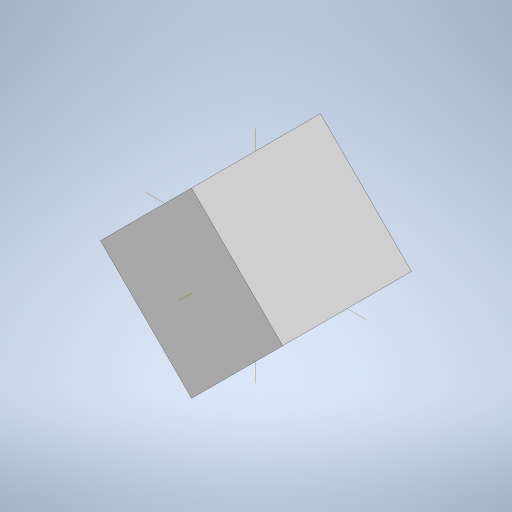
# Autodesk Inventor part: Cube
Saved by Autodesk Inventor 2023.1 (Build 271208000, 208)
## iProperties
Created: 2023-01-19
Part Number: Cube
Material: Generisch
Document SubType Name: Modeling
Designer: mehan
Density: 1 g/cm^3
Appearance: Vorgabe
Author: mehan
Autodesk Inventor part; units mm, degrees
ref_plane "YZ Plane" through (0, 0, 0) normal (1, 0, 0) x (0, 1, 0)
ref_plane "XZ Plane" through (0, 0, 0) normal (0, 1, 0) x (-1, 0, 0)
ref_plane "XY Plane" through (0, 0, 0) normal (0, 0, 1) x (1, 0, 0)
sketch "Skizze2" plane through (0, 0, 0) normal (0, 0, 1) x (1, 0, 0)
  line L0 (0, 0) -> (37.5, 0) construction
  line L1 (26.5165, 26.5165) -> (53.033, 0)
  line L2 (53.033, 0) -> (26.5165, -26.5165)
  line L3 (-26.5165, 26.5165) -> (0, 53.033)
  line L4 (0, 53.033) -> (26.5165, 26.5165)
  line L5 (-26.5165, 26.5165) -> (-53.033, 0)
  line L6 (-53.033, 0) -> (0, -53.033)
  line L7 (0, -53.033) -> (26.5165, -26.5165)
  dimension "d12" = 37.5
  dimension "d15" = 37.5
  constraints: 16 end point, 4 perpendicular, 1 horizontal, 1 point on line
  measures "d12" distance of L1.start L1.end
  measures "d15" distance of L3.start L5.end
extrude "Extrusion2" add sketch "Skizze2" along normal mid plane 75
